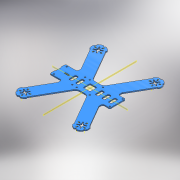
# Autodesk Inventor part: Base Plate
Saved by Autodesk Inventor 2018 (Build 220112000, 112)
## iProperties
Created: 2018-01-03
Part Number: Base Plate
Material: CFRP
Document SubType Name: Modeling
Designer: fbl92568
Mass: 45.8648 g
Surface Area: 302.598 cm^2
Volume: 32.0733 cm^3
Density: 1.43 g/cm^3
Appearance: Carbon Fiber
Author: fbl92568
Autodesk Inventor part; units mm, degrees
(part 1 of 2)
ref_plane "YZ Plane" through (0, 0, 0) normal (1, 0, 0) x (0, 1, 0)
ref_plane "XZ Plane" through (0, 0, 0) normal (0, 1, 0) x (-1, 0, 0)
ref_plane "XY Plane" through (0, 0, 0) normal (0, 0, 1) x (1, 0, 0)
sketch "Sketch1" plane through (0, 0, 0) normal (0, 0, 1) x (1, 0, 0)
  line L0 (-67.1964, 17.75) -> (63.6972, 17.75)
  line L1 (68.5, 12.9472) -> (68.5, 0)
  line L2 (-68.5, 8) -> (-68.5, 15.1428)
  line L3 (-68.5, 17.75) -> (0, 0) construction
  line L4 (68.5, 17.75) -> (0, 0) construction
  line L5 (-62.5, 14.75) -> (65.5, 14.75) construction
  line L6 (-89.2201, 0) -> (135.4294, 0) construction
  circle A0 centre (-62.5, 14.75) radius 1.525
  circle A1 centre (-20.5, 14.75) radius 1.525
  circle A2 centre (65.5, 14.75) radius 1.525
  arc A3 (68.5, 12.9472) -> (63.6972, 17.75) centre (65.5, 14.75) ccw
  line L7 (-68.5, 8) -> (-67, 5.5)
  line L8 (-67, 5.5) -> (-67, 0)
  line L9 (-67.1964, 17.75) -> (-68.5, 15.1428)
  line L10 (-67.1964, -17.75) -> (63.6972, -17.75)
  line L11 (68.5, -12.9472) -> (68.5, 0)
  line L12 (-68.5, -8) -> (-68.5, -15.1428)
  line L13 (-68.5, -17.75) -> (0, 0) construction
  line L14 (68.5, -17.75) -> (0, 0) construction
  line L15 (-62.5, -14.75) -> (65.5, -14.75) construction
  circle A4 centre (-62.5, -14.75) radius 1.525
  circle A5 centre (-20.5, -14.75) radius 1.525
  circle A6 centre (65.5, -14.75) radius 1.525
  arc A7 (63.6972, -17.75) -> (68.5, -12.9472) centre (65.5, -14.75) ccw
  line L16 (-68.5, -8) -> (-67, -5.5)
  line L17 (-67, -5.5) -> (-67, 0)
  line L18 (-67.1964, -17.75) -> (-68.5, -15.1428)
  line L19 (-10, 15) -> (20, 15) construction
  circle A8 centre (-10, 15) radius 1.525
  circle A9 centre (20, 15) radius 1.525
  circle A10 centre (-10, -15) radius 1.525
  circle A11 centre (20, -15) radius 1.525
  point P0 (0, 0)
  dimension "d0" = 137
  dimension "d2" = 3.05
  dimension "d3" = 3.05
  dimension "d4" = 3.05
  dimension "d5" = 6
  dimension "d6" = 42
  dimension "d7" = 86
  dimension "d8" = 3
  dimension "d9" = 7
  dimension "d10" = 35.5
  dimension "d12" = 68.5
  dimension "d13" = 68.5
  dimension "d17" = 1.5
  dimension "d18" = 5.5
  dimension "d19" = 9.75
  dimension "d20" = 8
  dimension "d21" = 1.3036
  dimension "d22" = 2.6072
  dimension "d25" = 3.05
  dimension "d26" = 3.05
  dimension "d27" = 58.5
  dimension "d28" = 30
  dimension "d30" = 15
  constraints: 40 end point, 16 symmetric about line, 12 centre point, 10 coincident, 5 point on line, 4 point on circle, 3 horizontal, 2 perpendicular, 1 parallel, 6 other
  measures "d0" distance of L3.start L4.start
  measures "d2" diameter of A0
  measures "d3" diameter of A1
  measures "d4" diameter of A2
  measures "d5" distance from line of A0.centre L2
  measures "d6" distance of A1.centre A0.centre
  measures "d7" distance of A2.centre A1.centre
  measures "d8" distance between parallel lines of L0 L5
  measures "d9" diameter of A3
  measures "d10" diameter of L0 L6
  measures "d12" distance from line of L2 point (0, 0)
  measures "d13" distance from line of point (0, 0) L1
  measures "d17" distance from line of L3.start L8
  measures "d18" distance of L7.end L8.end
  measures "d19" distance of L2.start L3.start
  measures "d20" vertical distance of point (0, 0) L2.start
  measures "d21" distance from line of L2 L0.start
  measures "d22" distance from line of L2.end L0
  measures "d25" diameter of A8
  measures "d26" diameter of A9
  measures "d27" distance from line of L19.start L2
  measures "d28" distance of L19.start L19.end
  measures "d30" distance from line of L19 point (0, 0)
extrude "Extrusion1" add sketch "Sketch1" along normal blind 2.5
sketch "Sketch2" plane through (0, 0, 0) normal (0, 0, -1) x (-1, 0, 0)
  circle A0 centre (59.6069, -83.7723) radius 4
  circle A1 centre (-70.3931, -83.7723) radius 4
  line L0 (67.1964, -17.75) -> (-63.6972, -17.75) projected
  line L1 (67.1964, -17.75) -> (-63.6972, -17.75) projected
  line L2 (-52.264, -26.3718) -> (-81.6514, -77.2723)
  line L3 (-17.264, -17.75) -> (-59.1348, -90.2723)
  arc A2 (-81.6514, -77.2723) -> (-59.1348, -90.2723) centre (-70.3931, -83.7723) ccw
  line L4 (70.8652, -77.2723) -> (41.4778, -26.3718)
  line L5 (48.3486, -90.2723) -> (6.4778, -17.75)
  arc A3 (48.3486, -90.2723) -> (70.8652, -77.2723) centre (59.6069, -83.7723) ccw
  line L6 (41.4778, -26.3718) -> (41.4778, -17.75)
  line L7 (67.1964, -17.75) -> (-63.6972, -17.75) projected
  line L8 (41.4778, -17.75) -> (6.4778, -17.75)
  line L9 (-52.264, -26.3718) -> (-52.264, -17.75)
  line L10 (-52.264, -17.75) -> (-17.264, -17.75)
  line L11 (59.6069, -83.7723) -> (-70.3931, -83.7723)
  line L12 (-68.5, -12.9472) -> (-68.5, 12.9472) projected
  line L13 (41.4778, -26.3718) -> (36.5, -17.75) construction
  line L14 (68.5, -8) -> (68.5, -15.1428) projected
  line L15 (89.2201, 0) -> (-135.4294, 0) construction
  circle A4 centre (59.6069, 83.7723) radius 4
  circle A5 centre (-70.3931, 83.7723) radius 4
  line L16 (67.1964, 17.75) -> (-63.6972, 17.75)
  line L17 (67.1964, 17.75) -> (-63.6972, 17.75)
  line L18 (-52.264, 26.3718) -> (-81.6514, 77.2723)
  line L19 (-17.264, 17.75) -> (-59.1348, 90.2723)
  arc A6 (-59.1348, 90.2723) -> (-81.6514, 77.2723) centre (-70.3931, 83.7723) ccw
  line L20 (70.8652, 77.2723) -> (41.4778, 26.3718)
  line L21 (48.3486, 90.2723) -> (6.4778, 17.75)
  arc A7 (70.8652, 77.2723) -> (48.3486, 90.2723) centre (59.6069, 83.7723) ccw
  line L22 (41.4778, 26.3718) -> (41.4778, 17.75)
  line L23 (67.1964, 17.75) -> (-63.6972, 17.75)
  line L24 (41.4778, 17.75) -> (6.4778, 17.75)
  line L25 (-52.264, 26.3718) -> (-52.264, 17.75)
  line L26 (-52.264, 17.75) -> (-17.264, 17.75)
  line L27 (59.6069, 83.7723) -> (-70.3931, 83.7723)
  line L28 (41.4778, 26.3718) -> (36.5, 17.75) construction
  point P0 (0, 0)
  point P1 (0, 0)
  point P2 (68.5, 15.1428)
  point P3 (-83.3931, 83.7723)
  point P4 (72.6069, 83.7723)
  point P5 (59.6069, 96.7723)
  point P6 (59.6069, -96.7723)
  dimension "d44" = 8
  dimension "d45" = 8
  dimension "d52" = 60
  dimension "d53" = 26
  dimension "d55" = 60
  dimension "d56" = 26
  dimension "d58" = 35
  dimension "d59" = 35
  dimension "d60" = 130
  dimension "d61" = 13
  dimension "d62" = 13
  dimension "d63" = 66.0223
  dimension "d65" = 32
  dimension "d94" = 156
  dimension "d95" = 193.5446
  constraints: 44 end point, 20 symmetric about line, 12 point on circle, 8 centre point, 8 point on line, 5 coincident, 3 collinear, 3 parallel, 2 tangent, 1 perpendicular, 1 vertical, 10 other
  measures "d44" diameter of A0
  measures "d45" diameter of A1
  measures "d52" angle of L2 L0
  measures "d53" distance between parallel lines of L2 L3
  measures "d55" angle of L0 L4
  measures "d56" distance between parallel lines of L4 L5
  measures "d58" distance from line of L3.start L9
  measures "d59" distance from line of L5.end L6
  measures "d60" distance of A1.centre A0.centre
  measures "d61" distance from line of L4 A0.centre
  measures "d62" distance from line of L3 A1.centre
  measures "d63" distance between parallel lines of L11 L0
  measures "d65" distance from line of L14 L13.end
  measures "d94" distance of point (72.607, 83.772) point (-83.393, 83.772)
  measures "d95" distance of point (59.607, -96.772) point (59.607, 96.772)
extrude "Extrusion2" add sketch "Sketch2" against normal up to surface (2.5 mm away) contours L6 L4 A3 L5 L0 | L3 A2 L2 L9 L0 | L16 L21 A7 L20 L22 | L16 L25 L18 A6 L19
ref_plane "Work Plane1" through (-59.6069, 83.7723, 2.5) normal (0, 1, 0) x (0, 0, 1)
ref_plane "Work Plane2" through (70.3931, -83.7723, 0) normal (0, -1, 0) x (0, 0, 1)
ref_plane "Work Plane3" through (-59.6069, 83.7723, 2.5) normal (1, 0, 0) x (0, 0, 1)
ref_plane "Work Plane4" through (70.3931, 83.7723, 0) normal (1, 0, 0) x (0, 0, 1)
ref_plane "Work Plane5" through (-59.6069, 0, 2.5) normal (0, 1, 0) x (0, 0, 1)
ref_plane "Work Plane6" through (5.3931, 83.7723, 2.5) normal (1, 0, 0) x (0, 0, 1)
sketch "Sketch3" plane through (0, 0, 2.5) normal (0, 0, 1) x (1, 0, 0)
  line L0 (59.5, 8) -> (56.5, 8)
  line L1 (54.5, 6) -> (54.5, -6)
  line L2 (56.5, -8) -> (59.5, -8)
  line L3 (61.5, -6) -> (61.5, 6)
  line L4 (59.5, 8) -> (-80.0714, 8) construction
  line L5 (-80.0714, -8) -> (87.5757, -8) construction
  circle A0 centre (-59.6069, 83.7723) radius 4 construction
  circle A1 centre (70.3931, 83.7723) radius 4 construction
  circle A2 centre (-59.6069, -83.7723) radius 4 construction
  circle A3 centre (70.3931, -83.7723) radius 4 construction
  circle A4 centre (20, -15) radius 1.525 construction
  circle A5 centre (-10, -15) radius 1.525 construction
  circle A6 centre (20, 15) radius 1.525 construction
  circle A7 centre (-10, 15) radius 1.525 construction
  circle A8 centre (65.5, -14.75) radius 1.525 construction
  circle A9 centre (-20.5, -14.75) radius 1.525 construction
  circle A10 centre (-62.5, -14.75) radius 1.525 construction
  circle A11 centre (65.5, 14.75) radius 1.525 construction
  circle A12 centre (-20.5, 14.75) radius 1.525 construction
  circle A13 centre (-62.5, 14.75) radius 1.525 construction
  line L6 (63.6972, 17.75) -> (52.264, 17.75) construction
  line L7 (52.264, 26.3718) -> (52.264, 17.75) construction
  line L8 (81.6514, 77.2723) -> (52.264, 26.3718) construction
  arc A14 (81.6514, 77.2723) -> (59.1348, 90.2723) centre (70.3931, 83.7723) ccw construction
  line L9 (17.264, 17.75) -> (59.1348, 90.2723) construction
  line L10 (17.264, 17.75) -> (-6.4778, 17.75) construction
  line L11 (-48.3486, 90.2723) -> (-6.4778, 17.75) construction
  arc A15 (-48.3486, 90.2723) -> (-70.8652, 77.2723) centre (-59.6069, 83.7723) ccw construction
  line L12 (-41.4778, 26.3718) -> (-70.8652, 77.2723) construction
  line L13 (-41.4778, 17.75) -> (-41.4778, 26.3718) construction
  line L14 (-41.4778, 17.75) -> (-67.1964, 17.75) construction
  line L15 (-67.1964, 17.75) -> (-68.5, 15.1428) construction
  line L16 (-68.5, 15.1428) -> (-68.5, 8) construction
  line L17 (-68.5, 8) -> (-67, 5.5) construction
  line L18 (-67, 5.5) -> (-67, -5.5) construction
  line L19 (-67, -5.5) -> (-68.5, -8) construction
  line L20 (-68.5, -8) -> (-68.5, -15.1428) construction
  line L21 (-68.5, -15.1428) -> (-67.1964, -17.75) construction
  line L22 (-67.1964, -17.75) -> (-41.4778, -17.75) construction
  line L23 (-41.4778, -26.3718) -> (-41.4778, -17.75) construction
  line L24 (-70.8652, -77.2723) -> (-41.4778, -26.3718) construction
  arc A16 (-70.8652, -77.2723) -> (-48.3486, -90.2723) centre (-59.6069, -83.7723) ccw construction
  line L25 (-6.4778, -17.75) -> (-48.3486, -90.2723) construction
  line L26 (-6.4778, -17.75) -> (17.264, -17.75) construction
  line L27 (59.1348, -90.2723) -> (17.264, -17.75) construction
  arc A17 (59.1348, -90.2723) -> (81.6514, -77.2723) centre (70.3931, -83.7723) ccw construction
  line L28 (52.264, -26.3718) -> (81.6514, -77.2723) construction
  line L29 (52.264, -17.75) -> (52.264, -26.3718) construction
  line L30 (52.264, -17.75) -> (63.6972, -17.75) construction
  arc A18 (63.6972, -17.75) -> (68.5, -12.9472) centre (65.5, -14.75) ccw construction
  line L31 (68.5, -12.9472) -> (68.5, 12.9472) construction
  arc A19 (68.5, 12.9472) -> (63.6972, 17.75) centre (65.5, 14.75) ccw construction
  line L32 (44.5, 8) -> (41.5, 8)
  line L33 (39.5, 6) -> (39.5, -6)
  line L34 (41.5, -8) -> (44.5, -8)
  line L35 (46.5, -6) -> (46.5, 6)
  line L36 (29.5, 8) -> (26.5, 8)
  line L37 (24.5, 6) -> (24.5, -6)
  line L38 (26.5, -8) -> (29.5, -8)
  line L39 (31.5, -6) -> (31.5, 6)
  line L40 (68.5, -12.9472) -> (68.5, 12.9472) projected
  line L41 (11.5, 8) -> (-0.5, 8)
  line L42 (-2.5, 6) -> (-2.5, -6)
  line L43 (-0.5, -8) -> (11.5, -8)
  line L44 (13.5, -6) -> (13.5, 6)
  line L45 (-15.5, 8) -> (-18.5, 8)
  line L46 (-20.5, 6) -> (-20.5, -6)
  line L47 (-18.5, -8) -> (-15.5, -8)
  line L48 (-13.5, -6) -> (-13.5, 6)
  line L49 (-30.5, 8) -> (-33.5, 8)
  line L50 (-35.5, 6) -> (-35.5, -6)
  line L51 (-33.5, -8) -> (-30.5, -8)
  line L52 (-28.5, -6) -> (-28.5, 6)
  arc A20 (-43.5, -1.5) -> (-43.5, 1.5) centre (-43.5, 0) ccw
  arc A21 (-51.5, 1.5) -> (-51.5, -1.5) centre (-51.5, 0) ccw
  line L53 (-43.5, 1.5) -> (-51.5, 1.5)
  line L54 (-43.5, -1.5) -> (-51.5, -1.5)
  arc A22 (-33.5, 8) -> (-35.5, 6) centre (-33.5, 6) ccw
  arc A23 (-35.5, -6) -> (-33.5, -8) centre (-33.5, -6) ccw
  arc A24 (-28.5, 6) -> (-30.5, 8) centre (-30.5, 6) ccw
  arc A25 (-30.5, -8) -> (-28.5, -6) centre (-30.5, -6) ccw
  arc A26 (-20.5, -6) -> (-18.5, -8) centre (-18.5, -6) ccw
  arc A27 (-18.5, 8) -> (-20.5, 6) centre (-18.5, 6) ccw
  arc A28 (-13.5, 6) -> (-15.5, 8) centre (-15.5, 6) ccw
  arc A29 (-15.5, -8) -> (-13.5, -6) centre (-15.5, -6) ccw
  arc A30 (-2.5, -6) -> (-0.5, -8) centre (-0.5, -6) ccw
  arc A31 (-0.5, 8) -> (-2.5, 6) centre (-0.5, 6) ccw
  arc A32 (13.5, 6) -> (11.5, 8) centre (11.5, 6) ccw
  arc A33 (11.5, -8) -> (13.5, -6) centre (11.5, -6) ccw
  arc A34 (24.5, -6) -> (26.5, -8) centre (26.5, -6) ccw
  arc A35 (29.5, -8) -> (31.5, -6) centre (29.5, -6) ccw
  arc A36 (31.5, 6) -> (29.5, 8) centre (29.5, 6) ccw
  arc A37 (26.5, 8) -> (24.5, 6) centre (26.5, 6) ccw
  arc A38 (41.5, 8) -> (39.5, 6) centre (41.5, 6) ccw
  arc A39 (39.5, -6) -> (41.5, -8) centre (41.5, -6) ccw
  arc A40 (44.5, -8) -> (46.5, -6) centre (44.5, -6) ccw
  arc A41 (46.5, 6) -> (44.5, 8) centre (44.5, 6) ccw
  arc A42 (56.5, 8) -> (54.5, 6) centre (56.5, 6) ccw
  arc A43 (61.5, 6) -> (59.5, 8) centre (59.5, 6) ccw
  arc A44 (61.5, 6) -> (59.5, 8) centre (59.5, 6) ccw
  arc A45 (59.5, -8) -> (61.5, -6) centre (59.5, -6) ccw
  arc A46 (54.5, -6) -> (56.5, -8) centre (56.5, -6) ccw
  line L55 (74.3931, -90.7005) -> (66.3931, -76.8441) construction
  line L56 (75.2591, -90.2005) -> (67.2591, -76.3441)
  line L57 (65.5271, -77.3441) -> (73.5271, -91.2005)
  arc A47 (73.5271, -91.2005) -> (75.2591, -90.2005) centre (74.3931, -90.7005) ccw
  arc A48 (67.2591, -76.3441) -> (65.5271, -77.3441) centre (66.3931, -76.8441) ccw
  line L58 (77.3213, -79.7723) -> (63.4649, -87.7723) construction
  line L59 (76.8213, -78.9063) -> (62.9649, -86.9063)
  line L60 (63.9649, -88.6383) -> (77.8213, -80.6383)
  arc A49 (77.8213, -80.6383) -> (76.8213, -78.9063) centre (77.3213, -79.7723) ccw
  arc A50 (62.9649, -86.9063) -> (63.9649, -88.6383) centre (63.4649, -87.7723) ccw
  line L61 (70.3931, -83.7723) -> (66.2497, -99.2356) construction
  line L62 (59.1348, -90.2723) -> (17.264, -17.75) projected
  line L63 (67.8049, -93.4316) -> (68.3226, -91.4997) construction
  line L64 (69.0123, -93.7551) -> (69.53, -91.8232)
  line L65 (67.1152, -91.1762) -> (66.5975, -93.108)
  arc A51 (66.5975, -93.108) -> (69.0123, -93.7551) centre (67.8049, -93.4316) ccw
  arc A52 (69.53, -91.8232) -> (67.1152, -91.1762) centre (68.3226, -91.4997) ccw
  arc A53 (62.3422, -82.9092) -> (62.9892, -80.4943) centre (62.6657, -81.7018) ccw
  line L66 (62.9892, -80.4943) -> (61.0574, -79.9767)
  line L67 (60.7339, -81.1841) -> (62.6657, -81.7018) construction
  line L68 (60.4103, -82.3915) -> (62.3422, -82.9092)
  arc A54 (61.0574, -79.9767) -> (60.4103, -82.3915) centre (60.7339, -81.1841) ccw
  arc A55 (71.2563, -75.7214) -> (73.6711, -76.3684) centre (72.4637, -76.0449) ccw
  line L69 (73.6711, -76.3684) -> (74.1887, -74.4366)
  line L70 (72.9813, -74.113) -> (72.4637, -76.0449) construction
  line L71 (71.7739, -73.7895) -> (71.2563, -75.7214)
  arc A56 (74.1887, -74.4366) -> (71.7739, -73.7895) centre (72.9813, -74.113) ccw
  arc A57 (78.444, -84.6354) -> (77.797, -87.0503) centre (78.1205, -85.8429) ccw
  line L72 (77.797, -87.0503) -> (79.7288, -87.5679)
  line L73 (80.0524, -86.3605) -> (78.1205, -85.8429) construction
  line L74 (80.3759, -85.1531) -> (78.444, -84.6354)
  arc A58 (79.7288, -87.5679) -> (80.3759, -85.1531) centre (80.0524, -86.3605) ccw
  line L75 (5.3931, 142.1429) -> (5.3931, -142.1429) projected
  line L76 (-113.716, 0) -> (121.796, 0) projected
  circle A59 centre (70.3931, 83.7723) radius 4 construction
  arc A60 (81.6514, 77.2723) -> (59.1348, 90.2723) centre (70.3931, 83.7723) ccw construction
  line L77 (74.3931, 90.7005) -> (66.3931, 76.8441) construction
  line L78 (75.2591, 90.2005) -> (67.2591, 76.3441)
  line L79 (65.5271, 77.3441) -> (73.5271, 91.2005)
  arc A61 (75.2591, 90.2005) -> (73.5271, 91.2005) centre (74.3931, 90.7005) ccw
  arc A62 (65.5271, 77.3441) -> (67.2591, 76.3441) centre (66.3931, 76.8441) ccw
  line L80 (77.3213, 79.7723) -> (63.4649, 87.7723) construction
  line L81 (76.8213, 78.9063) -> (62.9649, 86.9063)
  line L82 (63.9649, 88.6383) -> (77.8213, 80.6383)
  arc A63 (76.8213, 78.9063) -> (77.8213, 80.6383) centre (77.3213, 79.7723) ccw
  arc A64 (63.9649, 88.6383) -> (62.9649, 86.9063) centre (63.4649, 87.7723) ccw
  line L83 (70.3931, 83.7723) -> (66.2497, 99.2356) construction
  line L84 (67.8049, 93.4316) -> (68.3226, 91.4997) construction
  line L85 (69.0123, 93.7551) -> (69.53, 91.8232)
  line L86 (67.1152, 91.1762) -> (66.5975, 93.108)
  arc A65 (69.0123, 93.7551) -> (66.5975, 93.108) centre (67.8049, 93.4316) ccw
  arc A66 (67.1152, 91.1762) -> (69.53, 91.8232) centre (68.3226, 91.4997) ccw
  arc A67 (62.9892, 80.4943) -> (62.3422, 82.9092) centre (62.6657, 81.7018) ccw
  line L87 (62.9892, 80.4943) -> (61.0574, 79.9767)
  line L88 (60.7339, 81.1841) -> (62.6657, 81.7018) construction
  line L89 (60.4103, 82.3915) -> (62.3422, 82.9092)
  arc A68 (60.4103, 82.3915) -> (61.0574, 79.9767) centre (60.7339, 81.1841) ccw
  arc A69 (73.6711, 76.3684) -> (71.2563, 75.7214) centre (72.4637, 76.0449) ccw
  line L90 (73.6711, 76.3684) -> (74.1887, 74.4366)
  line L91 (72.9813, 74.113) -> (72.4637, 76.0449) construction
  line L92 (71.7739, 73.7895) -> (71.2563, 75.7214)
  arc A70 (71.7739, 73.7895) -> (74.1887, 74.4366) centre (72.9813, 74.113) ccw
  arc A71 (77.797, 87.0503) -> (78.444, 84.6354) centre (78.1205, 85.8429) ccw
  line L93 (77.797, 87.0503) -> (79.7288, 87.5679)
  line L94 (80.0524, 86.3605) -> (78.1205, 85.8429) construction
  line L95 (80.3759, 85.1531) -> (78.444, 84.6354)
  arc A72 (80.3759, 85.1531) -> (79.7288, 87.5679) centre (80.0524, 86.3605) ccw
  circle A73 centre (-59.6069, 83.7723) radius 4 construction
  circle A74 centre (-59.6069, -83.7723) radius 4 construction
  arc A75 (-48.3486, 90.2723) -> (-70.8652, 77.2723) centre (-59.6069, 83.7723) ccw construction
  arc A76 (-70.8652, -77.2723) -> (-48.3486, -90.2723) centre (-59.6069, -83.7723) ccw construction
  line L96 (-63.6069, -90.7005) -> (-55.6069, -76.8441) construction
  line L97 (-64.4729, -90.2005) -> (-56.4729, -76.3441)
  line L98 (-54.7409, -77.3441) -> (-62.7409, -91.2005)
  arc A77 (-64.4729, -90.2005) -> (-62.7409, -91.2005) centre (-63.6069, -90.7005) ccw
  arc A78 (-54.7409, -77.3441) -> (-56.4729, -76.3441) centre (-55.6069, -76.8441) ccw
  line L99 (-66.5351, -79.7723) -> (-52.6787, -87.7723) construction
  line L100 (-66.0351, -78.9063) -> (-52.1787, -86.9063)
  line L101 (-53.1787, -88.6383) -> (-67.0351, -80.6383)
  arc A79 (-66.0351, -78.9063) -> (-67.0351, -80.6383) centre (-66.5351, -79.7723) ccw
  arc A80 (-53.1787, -88.6383) -> (-52.1787, -86.9063) centre (-52.6787, -87.7723) ccw
  line L102 (-59.6069, -83.7723) -> (-55.4635, -99.2356) construction
  line L103 (-57.0187, -93.4316) -> (-57.5363, -91.4997) construction
  line L104 (-58.2261, -93.7551) -> (-58.7437, -91.8232)
  line L105 (-56.3289, -91.1762) -> (-55.8113, -93.108)
  arc A81 (-58.2261, -93.7551) -> (-55.8113, -93.108) centre (-57.0187, -93.4316) ccw
  arc A82 (-56.3289, -91.1762) -> (-58.7437, -91.8232) centre (-57.5363, -91.4997) ccw
  arc A83 (-52.203, -80.4943) -> (-51.556, -82.9092) centre (-51.8795, -81.7018) ccw
  line L106 (-52.203, -80.4943) -> (-50.2712, -79.9767)
  line L107 (-49.9476, -81.1841) -> (-51.8795, -81.7018) construction
  line L108 (-49.6241, -82.3915) -> (-51.556, -82.9092)
  arc A84 (-49.6241, -82.3915) -> (-50.2712, -79.9767) centre (-49.9476, -81.1841) ccw
  arc A85 (-62.8848, -76.3684) -> (-60.47, -75.7214) centre (-61.6774, -76.0449) ccw
  line L109 (-62.8848, -76.3684) -> (-63.4025, -74.4366)
  line L110 (-62.1951, -74.113) -> (-61.6774, -76.0449) construction
  line L111 (-60.9877, -73.7895) -> (-60.47, -75.7214)
  arc A86 (-60.9877, -73.7895) -> (-63.4025, -74.4366) centre (-62.1951, -74.113) ccw
  arc A87 (-67.0108, -87.0503) -> (-67.6578, -84.6354) centre (-67.3343, -85.8429) ccw
  line L112 (-67.0108, -87.0503) -> (-68.9426, -87.5679)
  line L113 (-69.2661, -86.3605) -> (-67.3343, -85.8429) construction
  line L114 (-69.5897, -85.1531) -> (-67.6578, -84.6354)
  arc A88 (-69.5897, -85.1531) -> (-68.9426, -87.5679) centre (-69.2661, -86.3605) ccw
  arc A89 (-55.8113, 93.108) -> (-58.2261, 93.7551) centre (-57.0187, 93.4316) ccw
  line L115 (-57.0187, 93.4316) -> (-57.5363, 91.4997) construction
  line L116 (-58.2261, 93.7551) -> (-58.7437, 91.8232)
  line L117 (-56.3289, 91.1762) -> (-55.8113, 93.108)
  arc A90 (-58.7437, 91.8232) -> (-56.3289, 91.1762) centre (-57.5363, 91.4997) ccw
  line L118 (-59.6069, 83.7723) -> (-55.4635, 99.2356) construction
  arc A91 (-52.1787, 86.9063) -> (-53.1787, 88.6383) centre (-52.6787, 87.7723) ccw
  circle A92 centre (-59.6069, 83.7723) radius 4 construction
  arc A93 (-48.3486, 90.2723) -> (-70.8652, 77.2723) centre (-59.6069, 83.7723) ccw construction
  line L119 (-53.1787, 88.6383) -> (-67.0351, 80.6383)
  line L120 (-66.5351, 79.7723) -> (-52.6787, 87.7723) construction
  line L121 (-66.0351, 78.9063) -> (-52.1787, 86.9063)
  arc A94 (-51.556, 82.9092) -> (-52.203, 80.4943) centre (-51.8795, 81.7018) ccw
  line L122 (-52.203, 80.4943) -> (-50.2712, 79.9767)
  arc A95 (-67.0351, 80.6383) -> (-66.0351, 78.9063) centre (-66.5351, 79.7723) ccw
  arc A96 (-56.4729, 76.3441) -> (-54.7409, 77.3441) centre (-55.6069, 76.8441) ccw
  line L123 (-54.7409, 77.3441) -> (-62.7409, 91.2005)
  line L124 (-63.6069, 90.7005) -> (-55.6069, 76.8441) construction
  arc A97 (-62.7409, 91.2005) -> (-64.4729, 90.2005) centre (-63.6069, 90.7005) ccw
  line L125 (-64.4729, 90.2005) -> (-56.4729, 76.3441)
  arc A98 (-68.9426, 87.5679) -> (-69.5897, 85.1531) centre (-69.2661, 86.3605) ccw
  arc A99 (-50.2712, 79.9767) -> (-49.6241, 82.3915) centre (-49.9476, 81.1841) ccw
  line L126 (-49.9476, 81.1841) -> (-51.8795, 81.7018) construction
  line L127 (-49.6241, 82.3915) -> (-51.556, 82.9092)
  line L128 (-60.9877, 73.7895) -> (-60.47, 75.7214)
  line L129 (-62.1951, 74.113) -> (-61.6774, 76.0449) construction
  arc A100 (-63.4025, 74.4366) -> (-60.9877, 73.7895) centre (-62.1951, 74.113) ccw
  arc A101 (-60.47, 75.7214) -> (-62.8848, 76.3684) centre (-61.6774, 76.0449) ccw
  line L130 (-62.8848, 76.3684) -> (-63.4025, 74.4366)
  arc A102 (-67.6578, 84.6354) -> (-67.0108, 87.0503) centre (-67.3343, 85.8429) ccw
  line L131 (-67.0108, 87.0503) -> (-68.9426, 87.5679)
  line L132 (-69.2661, 86.3605) -> (-67.3343, 85.8429) construction
  line L133 (-69.5897, 85.1531) -> (-67.6578, 84.6354)
  point P0 (0, 0)
  point P1 (61.5, 8)
  point P2 (54.5, 8)
  point P3 (46.5, 8)
  point P4 (39.5, -8)
  point P5 (31.5, 8)
  point P6 (24.5, -8)
  point P7 (13.5, 8)
  point P8 (-2.5, -8)
  point P9 (-13.5, 8)
  point P10 (-20.5, -8)
  point P11 (-28.5, 8)
  point P12 (-35.5, -8)
  point P13 (68.0637, -92.4656)
  point P14 (61.6998, -81.4429)
  point P15 (72.7225, -75.079)
  point P16 (79.0864, -86.1017)
  point P17 (68.0637, 92.4656)
  point P18 (61.6998, 81.4429)
  point P19 (72.7225, 75.079)
  point P20 (79.0864, 86.1017)
  point P21 (-57.2775, -92.4656)
  point P22 (-50.9136, -81.4429)
  point P23 (-61.9363, -75.079)
  point P24 (-68.3002, -86.1017)
  point P25 (-50.9136, 81.4429)
  point P26 (-57.2775, 92.4656)
  point P27 (-61.9363, 75.079)
  point P28 (-68.3002, 86.1017)
  dimension "d68" = 16
  dimension "d69" = 8
  dimension "d70" = 7
  dimension "d71" = 7
  dimension "d72" = 22
  dimension "d73" = 7
  dimension "d74" = 37
  dimension "d75" = 7
  dimension "d76" = 55
  dimension "d77" = 16
  dimension "d78" = 82
  dimension "d79" = 7
  dimension "d80" = 97
  dimension "d81" = 7
  dimension "d82" = 112
  dimension "d83" = 3
  dimension "d84" = 3
  dimension "d85" = 8
  dimension "d86" = 2
  dimension "d87" = 2
  dimension "d88" = 2
  dimension "d89" = 2
  dimension "d90" = 2
  dimension "d91" = 2
  dimension "d99" = 2
  dimension "d100" = 2
  dimension "d101" = 8
  dimension "d102" = 8
  dimension "d104" = 45
  dimension "d105" = 2.5
  dimension "d106" = 8
  dimension "d107" = 1
  dimension "d110" = 360
  constraints: 256 end point, 158 point on circle, 140 symmetric about line, 83 centre point, 64 tangent, 43 point on line, 19 equal radius, 17 parallel, 8 horizontal, 7 perpendicular, 3 midpoint, 2 coincident, 2 collinear, 94 other
  measures "d68" distance between parallel lines of L5 L4
  measures "d69" distance from line of point (0, 0) L4
  measures "d70" distance between parallel lines of L31 L3
  measures "d71" distance of point (61.5, 8) point (54.5, 8)
  measures "d72" distance between parallel lines of L31 L35
  measures "d73" distance between parallel lines of L35 L33
  measures "d74" distance between parallel lines of L39 L40
  measures "d75" distance between parallel lines of L39 L37
  measures "d76" distance between parallel lines of L44 L31
  measures "d77" distance between parallel lines of L42 L44
  measures "d78" distance between parallel lines of L31 L48
  measures "d79" distance between parallel lines of L46 L48
  measures "d80" distance between parallel lines of L52 L31
  measures "d81" distance between parallel lines of L52 L50
  measures "d82" distance from line of L31 A20.centre
  measures "d83" diameter of A20
  measures "d84" diameter of A21
  measures "d85" distance of A21.centre A20.centre
  measures "d86" radius of A22
  measures "d87" radius of A24
  measures "d88" radius of A27
  measures "d89" radius of A28
  measures "d90" radius of A29
  measures "d91" radius of A36
  measures "d99" diameter of A48
  measures "d100" diameter of A50
  measures "d101" distance of L55.end A3.centre
  measures "d102" distance of L61.start L58.end
  measures "d104" angle of L61 L58
  measures "d105" diameter of A52
  measures "d106" distance of L63.end A3.centre
  measures "d107" distance of L63.end point (68.064, -92.466)
extrude "Extrusion3" cut sketch "Sketch3" against normal through all
fillet "Fillet1" radius 4 4 edges at (-41.4778, -17.75, 1.25) (-41.4778, 17.75, 1.25) (52.264, 17.75, 1.25) (52.264, -17.75, 1.25)
fillet "Fillet1" radius 10 4 edges at (-6.4778, -17.75, 1.25) (17.264, -17.75, 1.25) (-6.4778, 17.75, 1.25) (17.264, 17.75, 1.25)
fillet "Fillet2" radius 1 12 edges at (52.264, -26.3718, 1.25) (52.264, 26.3718, 1.25) (-41.4778, 26.3718, 1.25) (-67.1964, 17.75, 1.25) (-68.5, 15.1428, 1.25) (-68.5, 8, 1.25) (-67, 5.5, 1.25) (-67, -5.5, 1.25) (-68.5, -8, 1.25) (-68.5, -15.1428, 1.25) (-67.1964, -17.75, 1.25) (-41.4778, -26.3718, 1.25)
sketch "Sketch4" plane through (0, 0, 2.5) normal (0, 0, 1) x (1, 0, 0)
  arc A0 (-67.4728, -17.1972) -> (-66.5784, -17.75) centre (-66.5784, -16.75) ccw projected
  line L0 (-66.5784, -17.75) -> (-45.4778, -17.75) projected
  arc A1 (-41.4778, -21.75) -> (-45.4778, -17.75) centre (-45.4778, -21.75) ccw projected
  line L1 (-41.4778, -26.1038) -> (-41.4778, -21.75) projected
  arc A2 (-41.6118, -26.6038) -> (-41.4778, -26.1038) centre (-42.4778, -26.1038) ccw projected
  line L2 (-70.8652, -77.2723) -> (-41.6118, -26.6038) projected
  arc A3 (-70.8652, -77.2723) -> (-48.3486, -90.2723) centre (-59.6069, -83.7723) ccw projected
  line L3 (-9.3645, -22.75) -> (-48.3486, -90.2723) projected
  arc A4 (-0.7043, -17.75) -> (-9.3645, -22.75) centre (-0.7043, -27.75) ccw projected
  line L4 (-0.7043, -17.75) -> (11.4905, -17.75) projected
  arc A5 (20.1508, -22.75) -> (11.4905, -17.75) centre (11.4905, -27.75) ccw projected
  line L5 (59.1348, -90.2723) -> (20.1508, -22.75) projected
  arc A6 (59.1348, -90.2723) -> (81.6514, -77.2723) centre (70.3931, -83.7723) ccw projected
  line L6 (52.398, -26.6038) -> (81.6514, -77.2723) projected
  arc A7 (52.264, -26.1038) -> (52.398, -26.6038) centre (53.264, -26.1038) ccw projected
  line L7 (52.264, -21.75) -> (52.264, -26.1038) projected
  arc A8 (56.264, -17.75) -> (52.264, -21.75) centre (56.264, -21.75) ccw projected
  line L8 (56.264, -17.75) -> (63.6972, -17.75) projected
  arc A9 (63.6972, -17.75) -> (68.5, -12.9472) centre (65.5, -14.75) ccw projected
  line L9 (68.5, -12.9472) -> (68.5, 12.9472) projected
  arc A10 (68.5, 12.9472) -> (63.6972, 17.75) centre (65.5, 14.75) ccw projected
  line L10 (63.6972, 17.75) -> (56.264, 17.75) projected
  arc A11 (52.264, 21.75) -> (56.264, 17.75) centre (56.264, 21.75) ccw projected
  line L11 (52.264, 26.1038) -> (52.264, 21.75) projected
  arc A12 (52.398, 26.6038) -> (52.264, 26.1038) centre (53.264, 26.1038) ccw projected
  line L12 (81.6514, 77.2723) -> (52.398, 26.6038) projected
  arc A13 (81.6514, 77.2723) -> (59.1348, 90.2723) centre (70.3931, 83.7723) ccw projected
  line L13 (20.1508, 22.75) -> (59.1348, 90.2723) projected
  arc A14 (11.4905, 17.75) -> (20.1508, 22.75) centre (11.4905, 27.75) ccw projected
  line L14 (11.4905, 17.75) -> (-0.7043, 17.75) projected
  arc A15 (-9.3645, 22.75) -> (-0.7043, 17.75) centre (-0.7043, 27.75) ccw projected
  line L15 (-48.3486, 90.2723) -> (-9.3645, 22.75) projected
  arc A16 (-48.3486, 90.2723) -> (-70.8652, 77.2723) centre (-59.6069, 83.7723) ccw projected
  line L16 (-41.6118, 26.6038) -> (-70.8652, 77.2723) projected
  arc A17 (-41.4778, 26.1038) -> (-41.6118, 26.6038) centre (-42.4778, 26.1038) ccw projected
  line L17 (-41.4778, 21.75) -> (-41.4778, 26.1038) projected
  arc A18 (-45.4778, 17.75) -> (-41.4778, 21.75) centre (-45.4778, 21.75) ccw projected
  line L18 (-45.4778, 17.75) -> (-66.5784, 17.75) projected
  arc A19 (-66.5784, 17.75) -> (-67.4728, 17.1972) centre (-66.5784, 16.75) ccw projected
  line L19 (-67.4728, 17.1972) -> (-68.3944, 15.3539) projected
  arc A20 (-68.3944, 15.3539) -> (-68.5, 14.9067) centre (-67.5, 14.9067) ccw projected
  line L20 (-68.5, 14.9067) -> (-68.5, 8.277) projected
  arc A21 (-68.5, 8.277) -> (-68.3575, 7.7625) centre (-67.5, 8.277) ccw projected
  line L21 (-68.3575, 7.7625) -> (-67.1425, 5.7375) projected
  arc A22 (-67, 5.223) -> (-67.1425, 5.7375) centre (-68, 5.223) ccw projected
  line L22 (-67, 5.223) -> (-67, -5.223) projected
  arc A23 (-67.1425, -5.7375) -> (-67, -5.223) centre (-68, -5.223) ccw projected
  line L23 (-67.1425, -5.7375) -> (-68.3575, -7.7625) projected
  arc A24 (-68.3575, -7.7625) -> (-68.5, -8.277) centre (-67.5, -8.277) ccw projected
  line L24 (-68.5, -8.277) -> (-68.5, -14.9067) projected
  arc A25 (-68.5, -14.9067) -> (-68.3944, -15.3539) centre (-67.5, -14.9067) ccw projected
  line L25 (-68.3944, -15.3539) -> (-67.4728, -17.1972) projected
  line L26 (-63.461, -82.7018) -> (-67.0351, -80.6383) projected
  arc A26 (-66.0351, -78.9063) -> (-67.0351, -80.6383) centre (-66.5351, -79.7723) ccw projected
  line L27 (-66.0351, -78.9063) -> (-62.461, -80.9698) projected
  arc A27 (-58.5364, -79.9182) -> (-62.461, -80.9698) centre (-59.6069, -83.7723) ccw projected
  line L28 (-58.5364, -79.9182) -> (-56.4729, -76.3441) projected
  arc A28 (-54.7409, -77.3441) -> (-56.4729, -76.3441) centre (-55.6069, -76.8441) ccw projected
  line L29 (-54.7409, -77.3441) -> (-56.8044, -80.9182) projected
  arc A29 (-55.7528, -84.8428) -> (-56.8044, -80.9182) centre (-59.6069, -83.7723) ccw projected
  line L30 (-55.7528, -84.8428) -> (-52.1787, -86.9063) projected
  arc A30 (-53.1787, -88.6383) -> (-52.1787, -86.9063) centre (-52.6787, -87.7723) ccw projected
  line L31 (-53.1787, -88.6383) -> (-56.7528, -86.5748) projected
  arc A31 (-60.6774, -87.6264) -> (-56.7528, -86.5748) centre (-59.6069, -83.7723) ccw projected
  line L32 (-60.6774, -87.6264) -> (-62.7409, -91.2005) projected
  arc A32 (-64.4729, -90.2005) -> (-62.7409, -91.2005) centre (-63.6069, -90.7005) ccw projected
  line L33 (-64.4729, -90.2005) -> (-62.4094, -86.6264) projected
  arc A33 (-63.461, -82.7018) -> (-62.4094, -86.6264) centre (-59.6069, -83.7723) ccw projected
  line L34 (-62.7409, 91.2005) -> (-60.6774, 87.6264) projected
  arc A34 (-56.7528, 86.5748) -> (-60.6774, 87.6264) centre (-59.6069, 83.7723) ccw projected
  line L35 (-56.7528, 86.5748) -> (-53.1787, 88.6383) projected
  arc A35 (-52.1787, 86.9063) -> (-53.1787, 88.6383) centre (-52.6787, 87.7723) ccw projected
  line L36 (-52.1787, 86.9063) -> (-55.7528, 84.8428) projected
  arc A36 (-56.8044, 80.9182) -> (-55.7528, 84.8428) centre (-59.6069, 83.7723) ccw projected
  line L37 (-56.8044, 80.9182) -> (-54.7409, 77.3441) projected
  arc A37 (-56.4729, 76.3441) -> (-54.7409, 77.3441) centre (-55.6069, 76.8441) ccw projected
  line L38 (-56.4729, 76.3441) -> (-58.5364, 79.9182) projected
  arc A38 (-62.461, 80.9698) -> (-58.5364, 79.9182) centre (-59.6069, 83.7723) ccw projected
  line L39 (-62.461, 80.9698) -> (-66.0351, 78.9063) projected
  arc A39 (-67.0351, 80.6383) -> (-66.0351, 78.9063) centre (-66.5351, 79.7723) ccw projected
  line L40 (-67.0351, 80.6383) -> (-63.461, 82.7018) projected
  arc A40 (-62.4094, 86.6264) -> (-63.461, 82.7018) centre (-59.6069, 83.7723) ccw projected
  line L41 (-62.4094, 86.6264) -> (-64.4729, 90.2005) projected
  arc A41 (-62.7409, 91.2005) -> (-64.4729, 90.2005) centre (-63.6069, 90.7005) ccw projected
  line L42 (67.5906, -80.9182) -> (65.5271, -77.3441) projected
  arc A42 (67.2591, -76.3441) -> (65.5271, -77.3441) centre (66.3931, -76.8441) ccw projected
  line L43 (67.2591, -76.3441) -> (69.3226, -79.9182) projected
  arc A43 (73.2472, -80.9698) -> (69.3226, -79.9182) centre (70.3931, -83.7723) ccw projected
  line L44 (73.2472, -80.9698) -> (76.8213, -78.9063) projected
  arc A44 (77.8213, -80.6383) -> (76.8213, -78.9063) centre (77.3213, -79.7723) ccw projected
  line L45 (77.8213, -80.6383) -> (74.2472, -82.7018) projected
  arc A45 (73.1956, -86.6264) -> (74.2472, -82.7018) centre (70.3931, -83.7723) ccw projected
  line L46 (73.1956, -86.6264) -> (75.2591, -90.2005) projected
  arc A46 (73.5271, -91.2005) -> (75.2591, -90.2005) centre (74.3931, -90.7005) ccw projected
  line L47 (73.5271, -91.2005) -> (71.4636, -87.6264) projected
  arc A47 (67.539, -86.5748) -> (71.4636, -87.6264) centre (70.3931, -83.7723) ccw projected
  line L48 (67.539, -86.5748) -> (63.9649, -88.6383) projected
  arc A48 (62.9649, -86.9063) -> (63.9649, -88.6383) centre (63.4649, -87.7723) ccw projected
  line L49 (62.9649, -86.9063) -> (66.539, -84.8428) projected
  arc A49 (67.5906, -80.9182) -> (66.539, -84.8428) centre (70.3931, -83.7723) ccw projected
  line L50 (63.9649, 88.6383) -> (67.539, 86.5748) projected
  arc A50 (71.4636, 87.6264) -> (67.539, 86.5748) centre (70.3931, 83.7723) ccw projected
  line L51 (71.4636, 87.6264) -> (73.5271, 91.2005) projected
  arc A51 (75.2591, 90.2005) -> (73.5271, 91.2005) centre (74.3931, 90.7005) ccw projected
  line L52 (75.2591, 90.2005) -> (73.1956, 86.6264) projected
  arc A52 (74.2472, 82.7018) -> (73.1956, 86.6264) centre (70.3931, 83.7723) ccw projected
  line L53 (74.2472, 82.7018) -> (77.8213, 80.6383) projected
  arc A53 (76.8213, 78.9063) -> (77.8213, 80.6383) centre (77.3213, 79.7723) ccw projected
  line L54 (76.8213, 78.9063) -> (73.2472, 80.9698) projected
  arc A54 (69.3226, 79.9182) -> (73.2472, 80.9698) centre (70.3931, 83.7723) ccw projected
  line L55 (69.3226, 79.9182) -> (67.2591, 76.3441) projected
  arc A55 (65.5271, 77.3441) -> (67.2591, 76.3441) centre (66.3931, 76.8441) ccw projected
  line L56 (65.5271, 77.3441) -> (67.5906, 80.9182) projected
  arc A56 (66.539, 84.8428) -> (67.5906, 80.9182) centre (70.3931, 83.7723) ccw projected
  line L57 (66.539, 84.8428) -> (62.9649, 86.9063) projected
  arc A57 (63.9649, 88.6383) -> (62.9649, 86.9063) centre (63.4649, 87.7723) ccw projected
  arc A58 (11.5, -8) -> (13.5, -6) centre (11.5, -6) ccw projected
  line L58 (11.5, -8) -> (-0.5, -8) projected
  arc A59 (-2.5, -6) -> (-0.5, -8) centre (-0.5, -6) ccw projected
  line L59 (-2.5, -6) -> (-2.5, 6) projected
  arc A60 (-0.5, 8) -> (-2.5, 6) centre (-0.5, 6) ccw projected
  line L60 (-0.5, 8) -> (11.5, 8) projected
  arc A61 (13.5, 6) -> (11.5, 8) centre (11.5, 6) ccw projected
  line L61 (13.5, 6) -> (13.5, -6) projected
  arc A62 (39.5, -6) -> (41.5, -8) centre (41.5, -6) ccw projected
  line L62 (39.5, -6) -> (39.5, 6) projected
  arc A63 (41.5, 8) -> (39.5, 6) centre (41.5, 6) ccw projected
  line L63 (41.5, 8) -> (44.5, 8) projected
  arc A64 (46.5, 6) -> (44.5, 8) centre (44.5, 6) ccw projected
  line L64 (46.5, 6) -> (46.5, -6) projected
  arc A65 (44.5, -8) -> (46.5, -6) centre (44.5, -6) ccw projected
  line L65 (44.5, -8) -> (41.5, -8) projected
  arc A66 (-20.5, -6) -> (-18.5, -8) centre (-18.5, -6) ccw projected
  line L66 (-20.5, -6) -> (-20.5, 6) projected
  arc A67 (-18.5, 8) -> (-20.5, 6) centre (-18.5, 6) ccw projected
  line L67 (-18.5, 8) -> (-15.5, 8) projected
  arc A68 (-13.5, 6) -> (-15.5, 8) centre (-15.5, 6) ccw projected
  line L68 (-13.5, 6) -> (-13.5, -6) projected
  arc A69 (-15.5, -8) -> (-13.5, -6) centre (-15.5, -6) ccw projected
  line L69 (-15.5, -8) -> (-18.5, -8) projected
  line L70 (-51.5, 1.5) -> (-43.5, 1.5) projected
  arc A70 (-43.5, -1.5) -> (-43.5, 1.5) centre (-43.5, 0) ccw projected
  line L71 (-43.5, -1.5) -> (-51.5, -1.5) projected
  arc A71 (-51.5, 1.5) -> (-51.5, -1.5) centre (-51.5, 0) ccw projected
  arc A72 (-67.6578, 84.6354) -> (-67.0108, 87.0503) centre (-67.3343, 85.8429) ccw projected
  line L72 (-67.6578, 84.6354) -> (-69.5897, 85.1531) projected
  arc A73 (-68.9426, 87.5679) -> (-69.5897, 85.1531) centre (-69.2661, 86.3605) ccw projected
  line L73 (-68.9426, 87.5679) -> (-67.0108, 87.0503) projected
  arc A74 (-63.4025, 74.4366) -> (-60.9877, 73.7895) centre (-62.1951, 74.113) ccw projected
  line L74 (-63.4025, 74.4366) -> (-62.8848, 76.3684) projected
  arc A75 (-60.47, 75.7214) -> (-62.8848, 76.3684) centre (-61.6774, 76.0449) ccw projected
  line L75 (-60.47, 75.7214) -> (-60.9877, 73.7895) projected
  arc A76 (-58.2261, -93.7551) -> (-55.8113, -93.108) centre (-57.0187, -93.4316) ccw projected
  line L76 (-58.2261, -93.7551) -> (-58.7437, -91.8232) projected
  arc A77 (-56.3289, -91.1762) -> (-58.7437, -91.8232) centre (-57.5363, -91.4997) ccw projected
  line L77 (-56.3289, -91.1762) -> (-55.8113, -93.108) projected
  arc A78 (-49.6241, -82.3915) -> (-50.2712, -79.9767) centre (-49.9476, -81.1841) ccw projected
  line L78 (-49.6241, -82.3915) -> (-51.556, -82.9092) projected
  arc A79 (-52.203, -80.4943) -> (-51.556, -82.9092) centre (-51.8795, -81.7018) ccw projected
  line L79 (-52.203, -80.4943) -> (-50.2712, -79.9767) projected
  arc A80 (77.797, 87.0503) -> (78.444, 84.6354) centre (78.1205, 85.8429) ccw projected
  line L80 (77.797, 87.0503) -> (79.7288, 87.5679) projected
  arc A81 (80.3759, 85.1531) -> (79.7288, 87.5679) centre (80.0524, 86.3605) ccw projected
  line L81 (80.3759, 85.1531) -> (78.444, 84.6354) projected
  arc A82 (67.1152, 91.1762) -> (69.53, 91.8232) centre (68.3226, 91.4997) ccw projected
  line L82 (67.1152, 91.1762) -> (66.5975, 93.108) projected
  arc A83 (69.0123, 93.7551) -> (66.5975, 93.108) centre (67.8049, 93.4316) ccw projected
  line L83 (69.0123, 93.7551) -> (69.53, 91.8232) projected
  arc A84 (71.2563, -75.7214) -> (73.6711, -76.3684) centre (72.4637, -76.0449) ccw projected
  line L84 (71.2563, -75.7214) -> (71.7739, -73.7895) projected
  arc A85 (74.1887, -74.4366) -> (71.7739, -73.7895) centre (72.9813, -74.113) ccw projected
  line L85 (74.1887, -74.4366) -> (73.6711, -76.3684) projected
  arc A86 (69.53, -91.8232) -> (67.1152, -91.1762) centre (68.3226, -91.4997) ccw projected
  line L86 (69.53, -91.8232) -> (69.0123, -93.7551) projected
  arc A87 (66.5975, -93.108) -> (69.0123, -93.7551) centre (67.8049, -93.4316) ccw projected
  line L87 (66.5975, -93.108) -> (67.1152, -91.1762) projected
  arc A88 (62.3422, -82.9092) -> (62.9892, -80.4943) centre (62.6657, -81.7018) ccw projected
  line L88 (62.3422, -82.9092) -> (60.4103, -82.3915) projected
  arc A89 (61.0574, -79.9767) -> (60.4103, -82.3915) centre (60.7339, -81.1841) ccw projected
  line L89 (61.0574, -79.9767) -> (62.9892, -80.4943) projected
  arc A90 (78.444, -84.6354) -> (77.797, -87.0503) centre (78.1205, -85.8429) ccw projected
  line L90 (78.444, -84.6354) -> (80.3759, -85.1531) projected
  arc A91 (79.7288, -87.5679) -> (80.3759, -85.1531) centre (80.0524, -86.3605) ccw projected
  line L91 (79.7288, -87.5679) -> (77.797, -87.0503) projected
  arc A92 (60.4103, 82.3915) -> (61.0574, 79.9767) centre (60.7339, 81.1841) ccw projected
  line L92 (60.4103, 82.3915) -> (62.3422, 82.9092) projected
  arc A93 (62.9892, 80.4943) -> (62.3422, 82.9092) centre (62.6657, 81.7018) ccw projected
  line L93 (62.9892, 80.4943) -> (61.0574, 79.9767) projected
  arc A94 (71.7739, 73.7895) -> (74.1887, 74.4366) centre (72.9813, 74.113) ccw projected
  line L94 (71.7739, 73.7895) -> (71.2563, 75.7214) projected
  arc A95 (73.6711, 76.3684) -> (71.2563, 75.7214) centre (72.4637, 76.0449) ccw projected
  line L95 (73.6711, 76.3684) -> (74.1887, 74.4366) projected
  arc A96 (-60.9877, -73.7895) -> (-63.4025, -74.4366) centre (-62.1951, -74.113) ccw projected
  line L96 (-60.9877, -73.7895) -> (-60.47, -75.7214) projected
  arc A97 (-62.8848, -76.3684) -> (-60.47, -75.7214) centre (-61.6774, -76.0449) ccw projected
  line L97 (-62.8848, -76.3684) -> (-63.4025, -74.4366) projected
  arc A98 (-69.5897, -85.1531) -> (-68.9426, -87.5679) centre (-69.2661, -86.3605) ccw projected
  line L98 (-69.5897, -85.1531) -> (-67.6578, -84.6354) projected
  arc A99 (-67.0108, -87.0503) -> (-67.6578, -84.6354) centre (-67.3343, -85.8429) ccw projected
  line L99 (-67.0108, -87.0503) -> (-68.9426, -87.5679) projected
  arc A100 (-50.2712, 79.9767) -> (-49.6241, 82.3915) centre (-49.9476, 81.1841) ccw projected
  line L100 (-50.2712, 79.9767) -> (-52.203, 80.4943) projected
  arc A101 (-51.556, 82.9092) -> (-52.203, 80.4943) centre (-51.8795, 81.7018) ccw projected
  line L101 (-51.556, 82.9092) -> (-49.6241, 82.3915) projected
  arc A102 (-58.7437, 91.8232) -> (-56.3289, 91.1762) centre (-57.5363, 91.4997) ccw projected
  line L102 (-58.7437, 91.8232) -> (-58.2261, 93.7551) projected
  arc A103 (-55.8113, 93.108) -> (-58.2261, 93.7551) centre (-57.0187, 93.4316) ccw projected
  line L103 (-55.8113, 93.108) -> (-56.3289, 91.1762) projected
  arc A104 (-33.5, 8) -> (-35.5, 6) centre (-33.5, 6) ccw projected
  line L104 (-33.5, 8) -> (-30.5, 8) projected
  arc A105 (-28.5, 6) -> (-30.5, 8) centre (-30.5, 6) ccw projected
  line L105 (-28.5, 6) -> (-28.5, -6) projected
  arc A106 (-30.5, -8) -> (-28.5, -6) centre (-30.5, -6) ccw projected
  line L106 (-30.5, -8) -> (-33.5, -8) projected
  arc A107 (-35.5, -6) -> (-33.5, -8) centre (-33.5, -6) ccw projected
  line L107 (-35.5, -6) -> (-35.5, 6) projected
  arc A108 (29.5, -8) -> (31.5, -6) centre (29.5, -6) ccw projected
  line L108 (29.5, -8) -> (26.5, -8) projected
  arc A109 (24.5, -6) -> (26.5, -8) centre (26.5, -6) ccw projected
  line L109 (24.5, -6) -> (24.5, 6) projected
  arc A110 (26.5, 8) -> (24.5, 6) centre (26.5, 6) ccw projected
  line L110 (26.5, 8) -> (29.5, 8) projected
  arc A111 (31.5, 6) -> (29.5, 8) centre (29.5, 6) ccw projected
  line L111 (31.5, 6) -> (31.5, -6) projected
  arc A112 (56.5, 8) -> (54.5, 6) centre (56.5, 6) ccw projected
  line L112 (56.5, 8) -> (59.5, 8) projected
  arc A113 (61.5, 6) -> (59.5, 8) centre (59.5, 6) ccw projected
  line L113 (61.5, 6) -> (61.5, -6) projected
  arc A114 (59.5, -8) -> (61.5, -6) centre (59.5, -6) ccw projected
  line L114 (59.5, -8) -> (56.5, -8) projected
  arc A115 (54.5, -6) -> (56.5, -8) centre (56.5, -6) ccw projected
  line L115 (54.5, -6) -> (54.5, 6) projected
  circle A116 centre (20, -15) radius 1.525 projected
  circle A117 centre (-10, -15) radius 1.525 projected
  circle A118 centre (20, 15) radius 1.525 projected
  circle A119 centre (-10, 15) radius 1.525 projected
  circle A120 centre (65.5, -14.75) radius 1.525 projected
  circle A121 centre (-20.5, -14.75) radius 1.525 projected
  circle A122 centre (-62.5, -14.75) radius 1.525 projected
  circle A123 centre (65.5, 14.75) radius 1.525 projected
  circle A124 centre (-20.5, 14.75) radius 1.525 projected
  circle A125 centre (-62.5, 14.75) radius 1.525 projected
  line L116 (121.2548, -83.7723) -> (-110.4686, -83.7723) projected
  line L117 (70.3931, 390.0401) -> (70.3931, -390.0401) projected
  line L118 (70.3931, -83.7723) -> (76.8931, -95.0306) construction
  line L119 (70.3931, -83.7723) -> (80.0419, -92.4844) construction
  arc A126 (59.1348, -90.2723) -> (81.6514, -77.2723) centre (70.3931, -83.7723) ccw projected
  line L120 (70.3931, -83.7723) -> (73.1137, -96.4844) construction
  arc A127 (73.1137, -96.4844) -> (80.0419, -92.4844) centre (70.3931, -83.7723) ccw construction
  arc A128 (73.5322, -98.4402) -> (81.5263, -93.8248) centre (70.3931, -83.7723) ccw
  arc A129 (72.6951, -94.5287) -> (78.5574, -91.1441) centre (70.3931, -83.7723) ccw
  arc A130 (72.6951, -94.5287) -> (73.5322, -98.4402) centre (73.1137, -96.4844) ccw
  arc A131 (81.5263, -93.8248) -> (78.5574, -91.1441) centre (80.0419, -92.4844) ccw
  line L121 (70.3931, -83.7723) -> (67.0285, -96.3293) construction
  line L122 (70.3931, -83.7723) -> (83.3931, -83.7723) construction
  line L123 (67.0285, -96.3293) -> (60.313, -91.9816) construction
  line L124 (60.313, -91.9816) -> (70.3931, -83.7723) construction
  line L125 (70.3931, -83.7723) -> (82.9501, -87.137) construction
  line L126 (70.3931, -83.7723) -> (83.3931, -83.7723) construction
  line L127 (82.9501, -87.137) -> (82.5426, -79.1473) construction
  line L128 (82.5426, -79.1473) -> (70.3931, -83.7723) construction
  arc A132 (60.313, -91.9816) -> (67.0285, -96.3293) centre (70.3931, -83.7723) ccw construction
  arc A133 (58.7623, -93.2445) -> (66.5108, -98.2612) centre (70.3931, -83.7723) ccw
  arc A134 (61.8638, -90.7186) -> (66.7941, -94.1669) centre (70.3931, -83.7723) ccw
  arc A135 (61.8638, -90.7186) -> (58.7623, -93.2445) centre (60.313, -91.9816) ccw
  arc A136 (66.5108, -98.2612) -> (68.1064, -94.6447) centre (67.0285, -96.3293) ccw
  arc A137 (82.9501, -87.137) -> (82.5426, -79.1473) centre (70.3931, -83.7723) ccw construction
  arc A138 (84.882, -87.6546) -> (84.4117, -78.4358) centre (70.3931, -83.7723) ccw
  arc A139 (81.1946, -85.8527) -> (80.6734, -79.8589) centre (70.3931, -83.7723) ccw
  arc A140 (80.9522, -87.2281) -> (84.882, -87.6546) centre (82.9501, -87.137) ccw
  arc A141 (84.4117, -78.4358) -> (80.6734, -79.8589) centre (82.5426, -79.1473) ccw
  line L129 (-110.4686, 0) -> (121.2548, 0) projected
  line L130 (5.3931, 390.0401) -> (5.3931, -390.0401) projected
  arc A142 (81.6514, 77.2723) -> (59.1348, 90.2723) centre (70.3931, 83.7723) ccw
  line L131 (70.3931, 83.7723) -> (76.8931, 95.0306) construction
  line L132 (70.3931, 83.7723) -> (80.0419, 92.4844) construction
  arc A143 (81.6514, 77.2723) -> (59.1348, 90.2723) centre (70.3931, 83.7723) ccw
  line L133 (70.3931, 83.7723) -> (73.1137, 96.4844) construction
  arc A144 (80.0419, 92.4844) -> (73.1137, 96.4844) centre (70.3931, 83.7723) ccw construction
  arc A145 (81.5263, 93.8248) -> (73.5322, 98.4402) centre (70.3931, 83.7723) ccw
  arc A146 (78.5574, 91.1441) -> (72.6951, 94.5287) centre (70.3931, 83.7723) ccw
  arc A147 (73.5322, 98.4402) -> (72.6951, 94.5287) centre (73.1137, 96.4844) ccw
  arc A148 (78.5574, 91.1441) -> (81.5263, 93.8248) centre (80.0419, 92.4844) ccw
  line L134 (70.3931, 83.7723) -> (67.0285, 96.3293) construction
  line L135 (70.3931, 83.7723) -> (83.3931, 83.7723) construction
  line L136 (67.0285, 96.3293) -> (60.313, 91.9816) construction
  line L137 (60.313, 91.9816) -> (70.3931, 83.7723) construction
  line L138 (70.3931, 83.7723) -> (82.9501, 87.137) construction
  line L139 (70.3931, 83.7723) -> (83.3931, 83.7723) construction
  line L140 (82.9501, 87.137) -> (82.5426, 79.1473) construction
  line L141 (82.5426, 79.1473) -> (70.3931, 83.7723) construction
  arc A149 (67.0285, 96.3293) -> (60.313, 91.9816) centre (70.3931, 83.7723) ccw construction
  arc A150 (66.5108, 98.2612) -> (58.7623, 93.2445) centre (70.3931, 83.7723) ccw
  arc A151 (66.7941, 94.1669) -> (61.8638, 90.7186) centre (70.3931, 83.7723) ccw
  arc A152 (58.7623, 93.2445) -> (61.8638, 90.7186) centre (60.313, 91.9816) ccw
  arc A153 (68.1064, 94.6447) -> (66.5108, 98.2612) centre (67.0285, 96.3293) ccw
  arc A154 (82.5426, 79.1473) -> (82.9501, 87.137) centre (70.3931, 83.7723) ccw construction
  arc A155 (84.4117, 78.4358) -> (84.882, 87.6546) centre (70.3931, 83.7723) ccw
  arc A156 (80.6734, 79.8589) -> (81.1946, 85.8527) centre (70.3931, 83.7723) ccw
  arc A157 (84.882, 87.6546) -> (80.9522, 87.2281) centre (82.9501, 87.137) ccw
  arc A158 (80.6734, 79.8589) -> (84.4117, 78.4358) centre (82.5426, 79.1473) ccw
  arc A159 (-48.3486, 90.2723) -> (-70.8652, 77.2723) centre (-59.6069, 83.7723) ccw
  arc A160 (-64.4729, -90.2005) -> (-62.7409, -91.2005) centre (-63.6069, -90.7005) ccw
  line L142 (-53.1787, 88.6383) -> (-56.7528, 86.5748)
  line L143 (-60.6774, 87.6264) -> (-62.7409, 91.2005)
  arc A161 (-62.7409, 91.2005) -> (-64.4729, 90.2005) centre (-63.6069, 90.7005) ccw
  line L144 (-64.4729, 90.2005) -> (-62.4094, 86.6264)
  arc A162 (-62.4094, 86.6264) -> (-63.461, 82.7018) centre (-59.6069, 83.7723) ccw
  line L145 (-63.461, 82.7018) -> (-67.0351, 80.6383)
  arc A163 (-67.0351, 80.6383) -> (-66.0351, 78.9063) centre (-66.5351, 79.7723) ccw
  line L146 (-66.0351, 78.9063) -> (-62.461, 80.9698)
  arc A164 (-52.1787, 86.9063) -> (-53.1787, 88.6383) centre (-52.6787, 87.7723) ccw
  arc A165 (-67.6578, 84.6354) -> (-67.0108, 87.0503) centre (-67.3343, 85.8429) ccw
  line L147 (-67.0108, 87.0503) -> (-68.9426, 87.5679)
  line L148 (-69.5897, 85.1531) -> (-67.6578, 84.6354)
  arc A166 (-58.7437, 91.8232) -> (-56.3289, 91.1762) centre (-57.5363, 91.4997) ccw
  line L149 (-56.3289, 91.1762) -> (-55.8113, 93.108)
  line L150 (-58.2261, 93.7551) -> (-58.7437, 91.8232)
  arc A167 (-56.3289, -91.1762) -> (-58.7437, -91.8232) centre (-57.5363, -91.4997) ccw
  line L151 (-58.7437, -91.8232) -> (-58.2261, -93.7551)
  arc A168 (-58.2261, -93.7551) -> (-55.8113, -93.108) centre (-57.0187, -93.4316) ccw
  line L152 (-55.8113, -93.108) -> (-56.3289, -91.1762)
  arc A169 (-60.47, 75.7214) -> (-62.8848, 76.3684) centre (-61.6774, 76.0449) ccw
  line L153 (-62.8848, 76.3684) -> (-63.4025, 74.4366)
  line L154 (-59.6069, 390.0401) -> (-59.6069, -390.0401)
  arc A170 (-69.2556, -92.4844) -> (-62.3274, -96.4844) centre (-59.6069, -83.7723) ccw construction
  arc A171 (-70.7401, -93.8248) -> (-62.746, -98.4402) centre (-59.6069, -83.7723) ccw
  arc A172 (-67.7712, -91.1441) -> (-61.9089, -94.5287) centre (-59.6069, -83.7723) ccw
  arc A173 (-62.746, -98.4402) -> (-61.9089, -94.5287) centre (-62.3274, -96.4844) ccw
  arc A174 (-67.7712, -91.1441) -> (-70.7401, -93.8248) centre (-69.2556, -92.4844) ccw
  line L155 (-56.2422, -96.3293) -> (-49.5268, -91.9816) construction
  line L156 (-72.1639, -87.137) -> (-71.7564, -79.1473) construction
  arc A175 (-56.2422, -96.3293) -> (-49.5268, -91.9816) centre (-59.6069, -83.7723) ccw construction
  arc A176 (-55.7246, -98.2612) -> (-47.976, -93.2445) centre (-59.6069, -83.7723) ccw
  arc A177 (-56.0078, -94.1669) -> (-51.0776, -90.7186) centre (-59.6069, -83.7723) ccw
  arc A178 (-47.976, -93.2445) -> (-51.0776, -90.7186) centre (-49.5268, -91.9816) ccw
  arc A179 (-57.3201, -94.6447) -> (-55.7246, -98.2612) centre (-56.2422, -96.3293) ccw
  arc A180 (-71.7564, -79.1473) -> (-72.1639, -87.137) centre (-59.6069, -83.7723) ccw construction
  arc A181 (-73.6255, -78.4358) -> (-74.0958, -87.6546) centre (-59.6069, -83.7723) ccw
  arc A182 (-69.8872, -79.8589) -> (-70.4084, -85.8527) centre (-59.6069, -83.7723) ccw
  arc A183 (-74.0958, -87.6546) -> (-70.166, -87.2281) centre (-72.1639, -87.137) ccw
  arc A184 (-69.8872, -79.8589) -> (-73.6255, -78.4358) centre (-71.7564, -79.1473) ccw